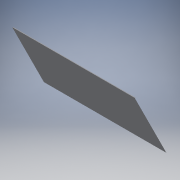
# Autodesk Inventor part: Seitenteil_Einbau
Saved by Autodesk Inventor 2016 (Build 200138000, 138)
## iProperties
Created: 2017-04-21
Part Number: Seitenteil_Einbau
Material: PVC, Unplasticized
Document SubType Name: Modeling
Designer: reinert
Density: 1.29 g/cm^3
Appearance: Smooth - White
Author: reinert
Autodesk Inventor part; units mm, degrees
ref_plane "YZ Plane" through (0, 0, 0) normal (1, 0, 0) x (0, 1, 0)
ref_plane "XZ Plane" through (0, 0, 0) normal (0, 1, 0) x (-1, 0, 0)
ref_plane "XY Plane" through (0, 0, 0) normal (0, 0, 1) x (1, 0, 0)
sketch "Sketch1" plane through (0, 0, 0) normal (0, 0, 1) x (1, 0, 0)
  line L0 (0, 0) -> (-462, 0)
  line L1 (-462, 0) -> (-462, 2)
  line L2 (-462, 2) -> (0, 2)
  line L3 (0, 2) -> (0, 0)
  dimension "d0" = 462
  dimension "d1" = 2
  constraints: 8 end point, 2 parallel, 1 horizontal, 1 perpendicular
  measures "d0" distance of L1.end L2.end
  measures "d1" distance of L2.end L0.start
extrude "Extrusion1" add sketch "Sketch1" along normal blind 90
body "Solid1"
